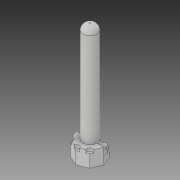
# Autodesk Inventor part: driver_handle
Saved by Autodesk Inventor 2019 (Build 230136000, 136)
## iProperties
Created: 2019-10-21
Part Number: driver_handle
Material: Generic
Document SubType Name: Modeling
Designer: devon
Density: 1 g/cm^3
Appearance: Default
Author: devon
Autodesk Inventor part; units mm, degrees
ref_plane "YZ Plane" through (0, 0, 0) normal (1, 0, 0) x (0, 1, 0)
ref_plane "XZ Plane" through (0, 0, 0) normal (0, 1, 0) x (-1, 0, 0)
ref_plane "XY Plane" through (0, 0, 0) normal (0, 0, 1) x (1, 0, 0)
sketch "Sketch1" plane through (0, 0, 0) normal (0, 1, 0) x (-1, 0, 0)
  line L0 (4.5, 1.988) -> (3.1372, -1.1754)
  line L1 (3.1372, -1.1754) -> (-0.0634, -2.4486)
  line L2 (-0.0634, -2.4486) -> (-3.2268, -1.0858)
  line L3 (-3.2268, -1.0858) -> (-4.5, 2.1147)
  line L4 (-4.5, 2.1147) -> (-3.1372, 5.2782)
  line L5 (-3.1372, 5.2782) -> (0.0634, 6.5514)
  line L6 (0.0634, 6.5514) -> (3.2268, 5.1885)
  line L7 (3.2268, 5.1885) -> (4.5, 1.988)
  point P0 (0, 0)
  point P1 (0, 2.0514)
  dimension "d0" = 9
  constraints: 16 end point, 17 other
  measures "d0" horizontal distance of L3.end L0.start
extrude "Extrusion1" add sketch "Sketch1" along normal blind 5
sketch "Sketch2" plane through (0, 5, 0) normal (0, 1, 0) x (1, 0, 0)
  line L0 (-3.1372, 1.1754) -> (-4.5, -1.988) projected
  line L1 (-4.5, -1.988) -> (-3.1372, 1.1754)
  line L2 (0.0634, 2.4486) -> (-3.1372, 1.1754) projected
  line L3 (-3.1372, 1.1754) -> (0.0634, 2.4486)
  line L4 (3.2268, 1.0858) -> (0.0634, 2.4486) projected
  line L5 (0.0634, 2.4486) -> (3.2268, 1.0858)
  line L6 (4.5, -2.1147) -> (3.2268, 1.0858) projected
  line L7 (3.2268, 1.0858) -> (4.5, -2.1147)
  line L8 (4.5, -2.1147) -> (-4.5, -1.988)
  point P0 (0, 0)
  constraints: 10 end point, 4 collinear
extrude "Extrusion2" cut sketch "Sketch2" against normal blind 2.5
sketch "Sketch3" plane through (0, 2.5, 0) normal (0, 1, 0) x (1, 0, 0)
  line L0 (-3.1372, 1.1754) -> (0.0634, 2.4486) projected
  circle A0 centre (-3.1372, 1.1754) radius 1
  circle A1 centre (0.0634, 2.4486) radius 1
  line L1 (0.0634, 2.4486) -> (3.2268, 1.0858) projected
  circle A2 centre (3.2268, 1.0858) radius 1
  point P0 (0, 0)
  dimension "d5" = 2
  dimension "d6" = 2
  dimension "d7" = 2
  constraints: 3 centre point, 1 coincident
  measures "d5" diameter of A0
  measures "d6" diameter of A1
  measures "d7" diameter of A2
extrude "Extrusion3" cut sketch "Sketch3" against normal blind 1
sketch "Sketch4" plane through (0, 5, 0) normal (0, 1, 0) x (1, 0, 0)
  line L0 (-3.2268, -5.1885) -> (-4.5, -1.988) projected
  circle A0 centre (-3.2268, -5.1885) radius 1
  line L1 (-0.0634, -6.5514) -> (-3.2268, -5.1885) projected
  circle A1 centre (-0.0634, -6.5514) radius 1
  line L2 (4.5, -2.1147) -> (3.1372, -5.2782) projected
  circle A2 centre (3.1372, -5.2782) radius 1
  point P0 (0, 0)
  dimension "d10" = 2
  dimension "d11" = 2
  dimension "d12" = 2
  constraints: 3 centre point
  measures "d10" diameter of A0
  measures "d11" diameter of A1
  measures "d12" diameter of A2
extrude "Extrusion4" cut sketch "Sketch4" against normal blind 1
sketch "Sketch5" plane through (0, 0, 0) normal (0, -1, 0) x (1, 0, 0)
  line L0 (4.5, 2.1147) -> (-4.5, 1.988) projected
  circle A0 centre (0, 2.0514) radius 0.875
  point P0 (0, 0)
  dimension "d15" = 1.75
  constraints: 1 centre point, 1 midpoint
  measures "d15" diameter of A0
extrude "Extrusion5" cut sketch "Sketch5" against normal through all
sketch "Sketch6" plane through (0, 2.5, 0) normal (0, 1, 0) x (1, 0, 0)
  arc A0 (0.8749, -2.0637) -> (-0.8749, -2.039) centre (0, -2.0514) ccw projected
  circle A1 centre (0, -2.0514) radius 2.25
  point P0 (0, 0)
  dimension "d18" = 4.5
  constraints: 1 centre point, 1 coincident
  measures "d18" diameter of A1
extrude "Extrusion6" add sketch "Sketch6" along normal blind 35
sketch "Sketch7" plane through (0, 2.5, 2.0514) normal (0, -1, 0) x (1, 0, 0)
  circle A0 centre (0, 0) radius 0.875
  point P0 (0, -2.0514)
  dimension "d23" = 1.75
  constraints: 1 centre point
  measures "d23" diameter of A0
extrude "Extrusion7" cut sketch "Sketch7" against normal blind 31
fillet "Fillet1" radius 2 1 edges at (-2.25, 37.5, 2.0514)
body "Solid1"
